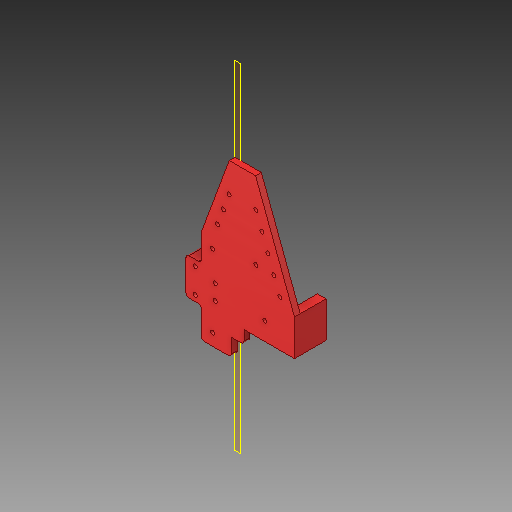
# Autodesk Inventor part: Neje_Support_Slider_Y
Saved by Autodesk Inventor 2019.4 (Build 234330000, 330)
## iProperties
Created: 2021-04-10
Part Number: Neje_Support_Slider_Y
Material: Generic
Document SubType Name: Modeling
Designer: diederichbenedict
Density: 1 g/cm^3
Appearance: Light Red
Author: diederichbenedict
Autodesk Inventor part; units mm, degrees
ref_plane "YZ Plane" through (0, 0, 0) normal (1, 0, 0) x (0, 1, 0)
ref_plane "Work Plane1" through (0, -17.1644, 1) normal (0, 0, 1) x (1, 0, 0)
sketch "Sketch1" plane through (0, -17.1644, 1) normal (0, 0, 1) x (1, 0, 0)
  circle A0 centre (25.1, 21.6249) radius 2.5 projected
  circle A1 centre (-23.15, 13.0749) radius 1.6 projected
  circle A2 centre (-9.28, 16.3749) radius 1.6 projected
  circle A3 centre (-11.1, -3.5751) radius 2.5 projected
  circle A4 centre (-11.1, 46.8249) radius 2.5 projected
  circle A5 centre (-9.28, 26.8749) radius 1.6 projected
  circle A6 centre (-23.15, 30.1749) radius 1.6 projected
  line L0 (-29.6, 10.9249) -> (-29.6, 32.3249) projected
  arc A7 (-29.6, 10.9249) -> (-27.6, 8.9249) centre (-27.6, 10.9249) ccw projected
  line L1 (-27.6, 8.9249) -> (-20.9, 8.9249) projected
  arc A8 (-18.9, 6.9249) -> (-20.9, 8.9249) centre (-20.9, 6.9249) ccw projected
  line L2 (-18.9, 6.9249) -> (-18.9, -9.8751) projected
  arc A9 (-18.9, -9.8751) -> (-16.9, -11.8751) centre (-16.9, -9.8751) ccw projected
  line L3 (-16.9, -11.8751) -> (0, -11.8751) projected
  arc A10 (0, -11.8751) -> (2, -9.8751) centre (0, -9.8751) ccw projected
  line L4 (2, -9.8751) -> (2, 0.1249) projected
  line L5 (2, 0.1249) -> (8.7, 0.1249) projected
  arc A11 (8.7, 0.1249) -> (10.7, 2.1249) centre (8.7, 2.1249) ccw projected
  line L6 (10.7, 2.1249) -> (10.7, 9.1249) projected
  line L7 (10.7, 9.1249) -> (45.7, 9.1249) projected
  line L8 (45.7, 34.1249) -> (45.7, 9.1249) projected
  line L9 (10.7, 34.1249) -> (45.7, 34.1249) projected
  line L10 (10.7, 41.1249) -> (10.7, 34.1249) projected
  arc A12 (10.7, 41.1249) -> (8.7, 43.1249) centre (8.7, 41.1249) ccw projected
  line L11 (2, 43.1249) -> (8.7, 43.1249) projected
  line L12 (2, 53.1249) -> (2, 43.1249) projected
  arc A13 (2, 53.1249) -> (0, 55.1249) centre (0, 53.1249) ccw projected
  line L13 (-16.9, 55.1249) -> (0, 55.1249) projected
  arc A14 (-16.9, 55.1249) -> (-18.9, 53.1249) centre (-16.9, 53.1249) ccw projected
  line L14 (-18.9, 36.3249) -> (-18.9, 53.1249) projected
  arc A15 (-20.9, 34.3249) -> (-18.9, 36.3249) centre (-20.9, 36.3249) ccw projected
  line L15 (-27.6, 34.3249) -> (-20.9, 34.3249) projected
  arc A16 (-27.6, 34.3249) -> (-29.6, 32.3249) centre (-27.6, 32.3249) ccw projected
  circle A17 centre (-11.1, -3.5751) radius 1.4
  circle A18 centre (-11.1, 46.8249) radius 1.4
  circle A19 centre (25.1, 21.6249) radius 1.4
  circle A20 centre (-23.15, 13.0749) radius 1.4
  circle A21 centre (-23.15, 30.1749) radius 1.4
  circle A22 centre (-9.28, 16.3749) radius 1.4
  circle A23 centre (-9.28, 26.8749) radius 1.4
  point P0 (0, 17.1644)
  dimension "d0" = 2.8
  dimension "d1" = 2.8
  dimension "d2" = 2.8
  dimension "d17" = 2.8
  dimension "d18" = 2.8
  dimension "d19" = 2.8
  dimension "d20" = 2.8
  constraints: 7 centre point, 7 coincident
  measures "d0" diameter of A17
  measures "d1" diameter of A18
  measures "d2" diameter of A19
  measures "d17" diameter of A20
  measures "d18" diameter of A21
  measures "d19" diameter of A22
  measures "d20" diameter of A23
extrude "Extrusion1" add sketch "Sketch1" along normal blind 4 contours A0 | A1 | A2 | A3 | A4 | A5 | A6 | L0 A16 L15 A15 L14 A14 L13 A13 L12 L11 A12 L10 L9 L8 L7 L6 A11 L5 L4 A10 L3 A9 L2 A8 L1 A7
sketch "Sketch2" plane through (0, -17.1644, 1) normal (0, 0, -1) x (-1, 0, 0)
  line L0 (29.6, 32.3249) -> (29.6, 10.9249) projected
  arc A0 (29.6, 32.3249) -> (27.6, 34.3249) centre (27.6, 32.3249) ccw projected
  line L1 (27.6, 34.3249) -> (20.9, 34.3249) projected
  arc A1 (18.9, 36.3249) -> (20.9, 34.3249) centre (20.9, 36.3249) ccw projected
  line L2 (18.9, 36.3249) -> (18.9, 53.1249) projected
  arc A2 (18.9, 53.1249) -> (16.9, 55.1249) centre (16.9, 53.1249) ccw projected
  line L3 (16.9, 55.1249) -> (0, 55.1249) projected
  arc A3 (0, 55.1249) -> (-2, 53.1249) centre (0, 53.1249) ccw projected
  line L4 (-2, 53.1249) -> (-2, 43.1249) projected
  line L5 (-2, 43.1249) -> (-8.7, 43.1249) projected
  arc A4 (-8.7, 43.1249) -> (-10.7, 41.1249) centre (-8.7, 41.1249) ccw projected
  line L6 (-10.7, 41.1249) -> (-10.7, 34.1249) projected
  line L7 (-10.7, 34.1249) -> (-45.7, 34.1249) projected
  line L8 (-45.7, 34.1249) -> (-45.7, 9.1249) projected
  line L9 (-10.7, 9.1249) -> (-45.7, 9.1249) projected
  line L10 (-10.7, 2.1249) -> (-10.7, 9.1249) projected
  arc A5 (-10.7, 2.1249) -> (-8.7, 0.1249) centre (-8.7, 2.1249) ccw projected
  line L11 (-2, 0.1249) -> (-8.7, 0.1249) projected
  line L12 (-2, -9.8751) -> (-2, 0.1249) projected
  arc A6 (-2, -9.8751) -> (0, -11.8751) centre (0, -9.8751) ccw projected
  line L13 (16.9, -11.8751) -> (0, -11.8751) projected
  arc A7 (16.9, -11.8751) -> (18.9, -9.8751) centre (16.9, -9.8751) ccw projected
  line L14 (18.9, 6.9249) -> (18.9, -9.8751) projected
  arc A8 (20.9, 8.9249) -> (18.9, 6.9249) centre (20.9, 6.9249) ccw projected
  line L15 (27.6, 8.9249) -> (20.9, 8.9249) projected
  arc A9 (27.6, 8.9249) -> (29.6, 10.9249) centre (27.6, 10.9249) ccw projected
  circle A10 centre (23.15, 13.0749) radius 1.6 projected
  circle A11 centre (9.28, 16.3749) radius 1.6 projected
  circle A12 centre (11.1, -3.5751) radius 2.5 projected
  circle A13 centre (11.1, 46.8249) radius 2.5 projected
  circle A14 centre (9.28, 26.8749) radius 1.6 projected
  circle A15 centre (23.15, 30.1749) radius 1.6 projected
  circle A16 centre (-25.1, 21.6249) radius 2.5 projected
  line L16 (20.9, 8.9249) -> (5.1431, 11.7032)
  line L17 (20.9, 8.9249) -> (36.9, 8.9249) construction
  line L18 (20.9, 34.3249) -> (5.1431, 31.5465)
  line L19 (20.9, 34.3249) -> (36.9, 34.3249) construction
  line L20 (5.1431, 31.5465) -> (5.1431, 11.7032)
  circle A17 centre (23.15, 30.1749) radius 1.4 projected
  circle A18 centre (23.15, 13.0749) radius 1.4 projected
  circle A19 centre (9.28, 16.3749) radius 1.4 projected
  circle A20 centre (9.28, 26.8749) radius 1.4 projected
  point P0 (0, 17.1644)
  dimension "d5" = 16
  dimension "d6" = 170
  dimension "d7" = 16
  dimension "d8" = 170
  constraints: 10 end point, 2 equal length, 2 horizontal
  measures "d5" distance of L15.end L16.end
  measures "d6" angle of L17 L16
  measures "d7" distance of L1.end L18.end
  measures "d8" angle of L18 L19
ref_plane "Work Plane2" through (-50.9629, -34.1365, -16.9) normal (0, 0, 1) x (0.751, -0.6603, 0)
extrude "Extrusion2" add sketch "Sketch2" along normal up to surface (17.9 mm away) contours L0 A9 L15 L16 L20 L18 L1 A0 | A10 | A11 | A14 | A15
sketch "Sketch3" plane through (-5.1431, -5.4612, 1) normal (1, 0, 0) x (0, 0, -1)
  line L0 (7.0236, 11.6716) -> (3.0236, 11.6716)
  line L1 (3.0236, 11.6716) -> (3.0236, 18.6716)
  line L2 (3.0236, 18.6716) -> (7.0236, 18.6716)
  line L3 (7.0236, 18.6716) -> (7.0236, 11.6716)
  line L4 (7.0236, 11.6716) -> (3.0236, 18.6716) construction
  line L5 (3.0236, 11.6716) -> (7.0236, 18.6716) construction
  line L6 (7.0236, 1.1716) -> (3.0236, 1.1716)
  line L7 (3.0236, 1.1716) -> (3.0236, 8.1716)
  line L8 (3.0236, 8.1716) -> (7.0236, 8.1716)
  line L9 (7.0236, 8.1716) -> (7.0236, 1.1716)
  line L10 (7.0236, 1.1716) -> (3.0236, 8.1716) construction
  line L11 (3.0236, 1.1716) -> (7.0236, 8.1716) construction
  line L12 (17.9, 3.2716) -> (-4, 3.2716) projected
  line L13 (17.9, 6.0716) -> (-4, 6.0716) projected
  line L14 (17.9, 13.7716) -> (-4, 13.7716) projected
  line L15 (17.9, 16.5716) -> (-4, 16.5716) projected
  point P0 (1, 5.4612)
  point P1 (5.0236, 15.1716)
  point P2 (5.0236, 4.6716)
  dimension "d11" = 4
  dimension "d12" = 7
  dimension "d13" = 4
  dimension "d14" = 7
  dimension "d22" = 1.4
  dimension "d23" = 1.4
  constraints: 24 end point, 4 midpoint, 4 parallel, 2 horizontal, 2 perpendicular
  measures "d11" distance of L1.end L2.end
  measures "d12" distance of L0.end L1.end
  measures "d13" distance of L7.end L8.end
  measures "d14" distance of L6.end L7.end
  measures "d22" distance from line of point (5.024, 4.672) L12
  measures "d23" distance from line of point (5.024, 15.172) L14
extrude "Extrusion3" cut sketch "Sketch3" against normal blind 8
sketch "Sketch4" plane through (-29.6, -6.2396, 5) normal (-1, 0, 0) x (0, 0, 1)
  line L0 (-19.9, 20.85) -> (-24.6, 20.85)
  line L1 (-19.9, 17.65) -> (-24.6, 17.65)
  line L2 (-24.6, 3.75) -> (-19.9, 3.75)
  line L3 (-24.6, 0.55) -> (-19.9, 0.55)
  line L4 (-12.9, 22.75) -> (-16.9, 22.75)
  line L5 (-16.9, 22.75) -> (-16.9, 15.75)
  line L6 (-16.9, 15.75) -> (-12.9, 15.75)
  line L7 (-12.9, 15.75) -> (-12.9, 22.75)
  line L8 (-12.9, 22.75) -> (-16.9, 15.75) construction
  line L9 (-16.9, 22.75) -> (-12.9, 15.75) construction
  line L10 (-16.9, -1.35) -> (-12.9, -1.35)
  line L11 (-12.9, -1.35) -> (-12.9, 5.65)
  line L12 (-12.9, 5.65) -> (-16.9, 5.65)
  line L13 (-16.9, 5.65) -> (-16.9, -1.35)
  line L14 (-16.9, -1.35) -> (-12.9, 5.65) construction
  line L15 (-12.9, -1.35) -> (-16.9, 5.65) construction
  line L16 (-21.9, 0) -> (-21.9, 21.4) projected
  point P0 (-5, 6.2396)
  point P1 (-14.9, 19.25)
  point P2 (-14.9, 2.15)
  dimension "d26" = 4
  dimension "d27" = 7
  dimension "d28" = 4
  dimension "d29" = 7
  dimension "d30" = 1.6
  dimension "d31" = 1.6
  dimension "d32" = 5
  dimension "d33" = 5
  constraints: 32 end point, 6 horizontal, 4 midpoint, 4 parallel, 2 perpendicular, 9 other
  measures "d26" distance of L6.end L5.end
  measures "d27" distance of L5.end L4.end
  measures "d28" distance of L12.end L11.end
  measures "d29" distance of L11.end L10.end
  measures "d30" distance from line of point (-14.9, 2.15) L2
  measures "d31" distance from line of point (-14.9, 19.25) L1
extrude "Extrusion4" cut sketch "Sketch4" against normal blind 10
sketch "Sketch5" plane through (0, -17.1644, 1) normal (0, 0, -1) x (-1, 0, 0)
  circle A0 centre (11.1, 46.8249) radius 1.4 projected
  circle A1 centre (11.1, -3.5751) radius 1.4 projected
  circle A2 centre (11.1, 46.8249) radius 3
  circle A3 centre (11.1, -3.5751) radius 3
  circle A4 centre (-25.1, 21.6249) radius 1.4 projected
  circle A5 centre (-25.1, 21.6249) radius 3
  point P0 (0, 17.1644)
  dimension "d36" = 6
  dimension "d37" = 6
  dimension "d38" = 6
  constraints: 3 centre point, 3 coincident
  measures "d36" diameter of A2
  measures "d37" diameter of A3
  measures "d38" diameter of A5
extrude "Extrusion5" add sketch "Sketch5" along normal blind 5
chamfer "Chamfer1" distance 4 angle 45 3 edges at (-8.1, 29.6604, 1) (-8.1, -20.7396, 1) (28.1, 4.4604, 1)
sketch "Sketch6" plane through (0, -17.1644, 1) normal (0, 0, -1) x (-1, 0, 0)
  line L0 (29.6, 32.3249) -> (29.6, 10.9249) projected
  arc A0 (29.6, 32.3249) -> (27.6, 34.3249) centre (27.6, 32.3249) ccw projected
  line L1 (27.6, 34.3249) -> (20.9, 34.3249) projected
  arc A1 (18.9, 36.3249) -> (20.9, 34.3249) centre (20.9, 36.3249) ccw projected
  line L2 (18.9, 36.3249) -> (18.9, 53.1249) projected
  arc A2 (18.9, 53.1249) -> (16.9, 55.1249) centre (16.9, 53.1249) ccw projected
  line L3 (16.9, 55.1249) -> (0, 55.1249) projected
  arc A3 (0, 55.1249) -> (-2, 53.1249) centre (0, 53.1249) ccw projected
  line L4 (-2, 53.1249) -> (-2, 43.1249) projected
  line L5 (-2, 43.1249) -> (-8.7, 43.1249) projected
  arc A4 (-8.7, 43.1249) -> (-10.7, 41.1249) centre (-8.7, 41.1249) ccw projected
  line L6 (-10.7, 41.1249) -> (-10.7, 34.1249) projected
  line L7 (-10.7, 34.1249) -> (-45.7, 34.1249) projected
  line L8 (-45.7, 34.1249) -> (-45.7, 9.1249) projected
  line L9 (-10.7, 9.1249) -> (-45.7, 9.1249) projected
  line L10 (-10.7, 2.1249) -> (-10.7, 9.1249) projected
  arc A5 (-10.7, 2.1249) -> (-8.7, 0.1249) centre (-8.7, 2.1249) ccw projected
  line L11 (-2, 0.1249) -> (-8.7, 0.1249) projected
  line L12 (-2, -9.8751) -> (-2, 0.1249) projected
  arc A6 (-2, -9.8751) -> (0, -11.8751) centre (0, -9.8751) ccw projected
  line L13 (16.9, -11.8751) -> (0, -11.8751) projected
  arc A7 (16.9, -11.8751) -> (18.9, -9.8751) centre (16.9, -9.8751) ccw projected
  line L14 (18.9, 6.9249) -> (18.9, -9.8751) projected
  arc A8 (20.9, 8.9249) -> (18.9, 6.9249) centre (20.9, 6.9249) ccw projected
  line L15 (27.6, 8.9249) -> (20.9, 8.9249) projected
  arc A9 (27.6, 8.9249) -> (29.6, 10.9249) centre (27.6, 10.9249) ccw projected
  circle A10 centre (23.15, 13.0749) radius 1.6 projected
  circle A11 centre (9.28, 16.3749) radius 1.6 projected
  circle A12 centre (11.1, -3.5751) radius 2.5 projected
  circle A13 centre (11.1, 46.8249) radius 2.5 projected
  circle A14 centre (9.28, 26.8749) radius 1.6 projected
  circle A15 centre (23.15, 30.1749) radius 1.6 projected
  circle A16 centre (-25.1, 21.6249) radius 2.5 projected
  line L16 (-10.7, 34.1249) -> (-45.7, 34.1249) projected
  line L17 (-45.7, 9.1249) -> (-10.7, 9.1249) projected
  line L18 (-45.7, 34.1249) -> (-39.7, 34.1249)
  line L19 (-39.7, 34.1249) -> (-39.7, 9.1249)
  line L20 (-39.7, 9.1249) -> (-45.7, 9.1249)
  line L21 (-45.7, 9.1249) -> (-45.7, 34.1249)
  point P0 (0, 17.1644)
  dimension "d44" = 6
  constraints: 8 end point, 2 parallel, 1 horizontal, 1 perpendicular, 1 point on line
  measures "d44" distance of L19.end L20.end
ref_plane "Work Plane3" through (-50.9629, -34.1365, -16.9) normal (0, 0, 1) x (0.751, -0.6603, 0)
extrude "Extrusion6" add sketch "Sketch6" along normal up to surface (17.9 mm away) contours L19 L9 L8 L7
chamfer "Chamfer2" distance 4 angle 45 1 edges at (39.7, 4.4604, 1)
sketch "Sketch7" plane through (0, -17.1644, 5) normal (0, 0, 1) x (1, 0, 0)
  circle A0 centre (-11.1, 46.8249) radius 1.4 projected
  circle A1 centre (-11.1, -3.5751) radius 1.4 projected
  circle A2 centre (25.1, 21.6249) radius 1.4 projected
  circle A3 centre (-23.15, 30.1749) radius 1.4 projected
  circle A4 centre (-9.28, 26.8749) radius 1.4 projected
  circle A5 centre (-9.28, 16.3749) radius 1.4 projected
  circle A6 centre (-23.15, 13.0749) radius 1.4 projected
  line L0 (-29.6, 32.3249) -> (-29.6, 10.9249) projected
  arc A7 (-29.6, 10.9249) -> (-27.6, 8.9249) centre (-27.6, 10.9249) ccw projected
  line L1 (-27.6, 8.9249) -> (-20.9, 8.9249) projected
  arc A8 (-18.9, 6.9249) -> (-20.9, 8.9249) centre (-20.9, 6.9249) ccw projected
  line L2 (-18.9, 6.9249) -> (-18.9, -9.8751) projected
  arc A9 (-18.9, -9.8751) -> (-16.9, -11.8751) centre (-16.9, -9.8751) ccw projected
  line L3 (-16.9, -11.8751) -> (0, -11.8751) projected
  arc A10 (0, -11.8751) -> (2, -9.8751) centre (0, -9.8751) ccw projected
  line L4 (2, -9.8751) -> (2, 0.1249) projected
  line L5 (2, 0.1249) -> (8.7, 0.1249) projected
  arc A11 (8.7, 0.1249) -> (10.7, 2.1249) centre (8.7, 2.1249) ccw projected
  line L6 (10.7, 2.1249) -> (10.7, 9.1249) projected
  line L7 (10.7, 9.1249) -> (45.7, 9.1249) projected
  line L8 (45.7, 9.1249) -> (45.7, 34.1249) projected
  line L9 (45.7, 34.1249) -> (10.7, 34.1249) projected
  line L10 (10.7, 34.1249) -> (10.7, 41.1249) projected
  arc A12 (10.7, 41.1249) -> (8.7, 43.1249) centre (8.7, 41.1249) ccw projected
  line L11 (8.7, 43.1249) -> (2, 43.1249) projected
  line L12 (2, 43.1249) -> (2, 53.1249) projected
  arc A13 (2, 53.1249) -> (0, 55.1249) centre (0, 53.1249) ccw projected
  line L13 (0, 55.1249) -> (-16.9, 55.1249) projected
  arc A14 (-16.9, 55.1249) -> (-18.9, 53.1249) centre (-16.9, 53.1249) ccw projected
  line L14 (-18.9, 53.1249) -> (-18.9, 36.3249) projected
  arc A15 (-20.9, 34.3249) -> (-18.9, 36.3249) centre (-20.9, 36.3249) ccw projected
  line L15 (-20.9, 34.3249) -> (-27.6, 34.3249) projected
  arc A16 (-27.6, 34.3249) -> (-29.6, 32.3249) centre (-27.6, 32.3249) ccw projected
  arc A17 (-16.9, 55.1249) -> (-18.9, 53.1249) centre (-16.9, 53.1249) ccw projected
  line L16 (-18.3142, 54.5391) -> (0.4, 105.5249)
  line L17 (0.4, 105.5249) -> (18.6828, 105.5249)
  line L18 (45.7, 9.1249) -> (45.7, 34.1249) projected
  line L19 (18.6828, 105.5249) -> (45.7, 34.1249)
  line L20 (45.7, 34.1249) -> (45.7, 9.1249)
  line L21 (45.7, 9.1249) -> (10.7, 9.1249)
  line L22 (15.9, 105.5249) -> (-23.6275, 105.5249) construction
  line L23 (-23.6275, 7.9249) -> (15.9, 7.9249) construction
  circle A18 centre (-14.28, 15.3749) radius 1.4 projected
  circle A19 centre (-14.28, 25.8749) radius 1.4 projected
  circle A20 centre (-12.7062, 62.1249) radius 1.4 projected
  circle A21 centre (-8.6687, 73.1249) radius 1.4 projected
  circle A22 centre (-4.6311, 84.1249) radius 1.4 projected
  circle A23 centre (-16.1, 45.8249) radius 6 projected
  line L24 (-23.6275, 7.9249) -> (-23.6275, 105.5249) projected
  line L25 (15.9, 7.9249) -> (15.9, 105.5249) projected
  point P0 (0, 17.1644)
  point P1 (45.7, 16.0196)
  point P2 (45.7, 15.9249)
  point P3 (15.9, 9.9249)
  constraints: 10 end point, 2 point on circle, 1 collinear, 1 horizontal, 1 perpendicular, 1 point on line
extrude "Extrusion7" add sketch "Sketch7" against normal up to surface (4 mm away) contours L16 L17 L25 L9 L10 A12 L11 L12 A13 L13 A14 | L17 L19 L9 L25 | A20 | A21 | A22
sketch "Sketch8" plane through (0, -17.1644, 1) normal (0, 0, -1) x (-1, 0, 0)
  line L0 (-35.7, 9.1249) -> (-35.7, 34.1249) projected
  line L1 (-35.7, 9.1249) -> (-10.7, 9.1249) projected
  line L2 (-10.7, 9.1249) -> (-10.7, 2.1249) projected
  arc A0 (-10.7, 2.1249) -> (-8.7, 0.1249) centre (-8.7, 2.1249) ccw projected
  line L3 (-8.7, 0.1249) -> (-2, 0.1249) projected
  line L4 (-2, 0.1249) -> (-2, -9.8751) projected
  arc A1 (-2, -9.8751) -> (0, -11.8751) centre (0, -9.8751) ccw projected
  line L5 (0, -11.8751) -> (16.9, -11.8751) projected
  arc A2 (16.9, -11.8751) -> (18.9, -9.8751) centre (16.9, -9.8751) ccw projected
  line L6 (18.9, -9.8751) -> (18.9, 6.9249) projected
  arc A3 (20.9, 8.9249) -> (18.9, 6.9249) centre (20.9, 6.9249) ccw projected
  line L7 (20.9, 8.9249) -> (5.1431, 11.7032) projected
  line L8 (5.1431, 11.7032) -> (5.1431, 31.5465) projected
  line L9 (5.1431, 31.5465) -> (20.9, 34.3249) projected
  arc A4 (18.9, 36.3249) -> (20.9, 34.3249) centre (20.9, 36.3249) ccw projected
  line L10 (18.9, 36.3249) -> (18.9, 53.1249) projected
  arc A5 (18.9, 53.1249) -> (18.3142, 54.5391) centre (16.9, 53.1249) ccw projected
  line L11 (18.3142, 54.5391) -> (-0.4, 105.5249) projected
  line L12 (-0.4, 105.5249) -> (-18.6828, 105.5249) projected
  line L13 (-18.6828, 105.5249) -> (-45.7, 34.1249) projected
  line L14 (-35.7, 34.1249) -> (-45.7, 34.1249) projected
  circle A6 centre (-25.1, 21.6249) radius 7 projected
  circle A7 centre (11.1, 46.8249) radius 7 projected
  circle A8 centre (11.1, -3.5751) radius 7 projected
  line L15 (-35.5669, 41.1249) -> (-13.8472, 98.5249)
  line L16 (-13.8472, 98.5249) -> (-5.2873, 98.5249)
  line L17 (-5.2873, 98.5249) -> (11.9, 51.6991)
  line L18 (11.9, 51.6991) -> (11.9, 39.8459)
  line L19 (11.9, 39.8459) -> (-1.8569, 37.4202)
  line L20 (-1.8569, 37.4202) -> (-1.8569, 5.8295)
  line L21 (-1.8569, 5.8295) -> (11.9, 3.4038)
  line L22 (11.9, 3.4038) -> (11.9, -4.8751)
  line L23 (11.9, -4.8751) -> (5, -4.8751)
  line L24 (5, -4.8751) -> (5, 7.1249)
  line L25 (5, 7.1249) -> (-3.7, 7.1249)
  line L26 (-3.7, 7.1249) -> (-3.7, 16.1249)
  line L27 (-3.7, 16.1249) -> (-28.7, 16.1249)
  line L28 (-28.7, 16.1249) -> (-28.7, 41.1249)
  line L29 (-28.7, 41.1249) -> (-35.5669, 41.1249)
  point P0 (0, 17.1644)
  point P1 (-18.9176, 85.1249)
  point P2 (-23.0799, 74.1249)
  point P3 (-27.2423, 63.1249)
  point P4 (-31.4046, 52.1249)
  point P5 (7.7062, 63.1249)
  point P6 (3.6687, 74.1249)
  point P7 (-0.3689, 85.1249)
  point P8 (-18.9176, 52.1249)
  dimension "d53" = 7
  dimension "d54" = 11
  dimension "d55" = 11
  dimension "d56" = 11
  dimension "d57" = 11
  constraints: 30 end point, 7 point on line, 1 coincident, 14 other
  measures "d53" distance between parallel lines of L13 L15
  measures "d54" vertical distance of point (-31.405, 52.125) point (-35.567, 41.125)
  measures "d55" vertical distance of point (-27.242, 63.125) point (-31.405, 52.125)
  measures "d56" vertical distance of point (-23.08, 74.125) point (-27.242, 63.125)
  measures "d57" vertical distance of point (-18.918, 85.125) point (-23.08, 74.125)
hole "Hole1" at (18.9176, 67.9604, 1) at (23.0799, 56.9604, 1) at (27.2423, 45.9604, 1) at (31.4046, 34.9604, 1) at (35.5669, 23.9604, 1) at (-7.7062, 45.9604, 1) at (-3.6687, 56.9604, 1) at (0.3689, 67.9604, 1) at (18.9176, 34.9604, 1) direction (0, 0, 1) diameter 2.8 end through all
body "Solid1"
